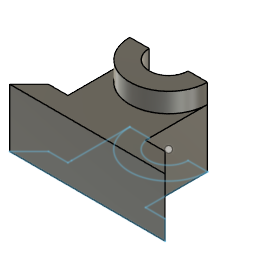
Ex4-lab1 (Autodesk Fusion 360 design; units mm, degrees)
part number: 2026-03-02-22-04-31-867
part number: 2026-03-02-22-37-46-315
Autodesk Fusion 360 part; units mm, degrees
sketch "Sketch1" plane through (0, 0, 0) normal (0, 0, 1) x (1, 0, 0) in component "Component"
sketch "Sketch1 (2)" plane through (0, 0, 0) normal (0, 0, 1) x (1, 0, 0)
sketch "Sketch2" plane through (0, 0, 0) normal (0, 0, 1) x (1, 0, 0) in component "Component"
  arc A0 (17.6425, 34.6248) -> (62.3575, 34.6248) centre (40, 35) ccw
  arc A1 (23.5355, 34.6248) -> (56.4645, 34.6248) centre (40, 36.7106) ccw
  line L0 (17.6425, 34.6248) -> (23.5355, 34.6248)
  line L1 (56.4645, 34.6248) -> (62.3575, 34.6248)
  constraint horizontal L0
  constraint collinear L0 L1
sketch "Sketch2 (2)" plane through (0, 0, 0) normal (0, 0, 1) x (1, 0, 0)
  line L0 (121.2193, 26.4028) -> (121.2193, 28.2696)
  line L1 (121.2193, 28.2696) -> (121.2193, 58.2696)
  line L2 (161.2193, 58.2696) -> (161.2193, 26.4028)
  line L3 (161.2193, 26.4028) -> (171.2193, 26.4028)
  line L4 (181.2193, 16.4028) -> (101.2193, 16.4028)
  line L5 (121.2193, 26.4028) -> (111.2193, 26.4028)
  line L6 (101.2193, 16.4028) -> (111.2193, 26.4028)
  line L7 (181.2193, 16.4028) -> (171.2193, 26.4028)
  arc A0 (131.2193, 58.2696) -> (151.2193, 58.2696) centre (141.2193, 58.2696) ccw
  arc A1 (121.2193, 58.2696) -> (161.2193, 58.2696) centre (141.2193, 58.2696) ccw
  line L8 (121.2193, 58.2696) -> (131.2193, 58.2696)
  line L9 (151.2193, 58.2696) -> (161.2193, 58.2696)
  dimension "d23" = 20
  dimension "d24" = 20
  dimension "d25" = 40
  dimension "d32" = 80
  dimension "d33" = 10
  constraint concentric A0 A1
  constraint perpendicular L1 L8
  constraint perpendicular L2 L3
  constraint perpendicular L0 L5
  constraint perpendicular L6 L7
  constraint perpendicular L2 L9
  measures "d23" distance of L1.end A0.centre
  measures "d24" diameter of A0
  measures "d25" diameter of A1
  measures "d32" distance of L4.start L4.end
  measures "d33" distance of L0.start L5.end
extrude "Extrude1" add sketch "Sketch2 (2)" along normal blind 40 contours A0 A1 L8 L9
extrude "Extrude2" add sketch "Sketch2 (2)" along normal blind 30 contours L0 L1 L2 L3 L4 L5 L6 L7 A1
component "Component" placed x (1, 0, 0) y (0, 1, 0) z (0, 0, 1) at (0, 0, 0)
